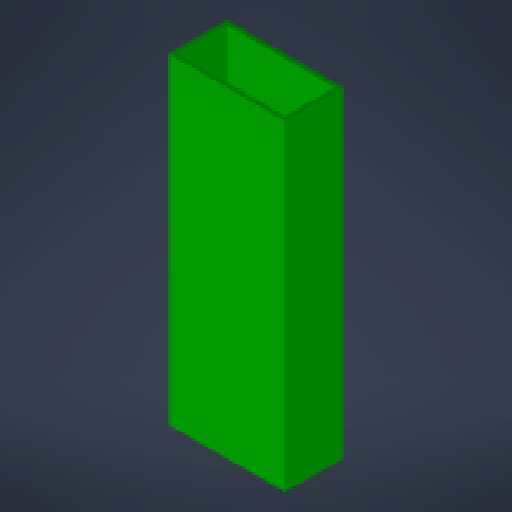
# Autodesk Inventor part: main axis
Saved by Autodesk Inventor 2024 (Build 280153000, 153)
## iProperties
Created: 2023-04-17
Part Number: main axis
Material: Типовые
Document SubType Name: Modeling
Designer: user
Density: 1 g/cm^3
Appearance: По умолчанию
Author: user
Autodesk Inventor part; units mm, degrees
ref_plane "YZ Plane" through (0, 0, 0) normal (1, 0, 0) x (0, 1, 0)
ref_plane "XZ Plane" through (0, 0, 0) normal (0, 1, 0) x (-1, 0, 0)
ref_plane "XY Plane" through (0, 0, 0) normal (0, 0, 1) x (1, 0, 0)
sketch "Эскиз1" plane through (0, 0, 0) normal (0, 0, 1) x (1, 0, 0)
  line L0 (0, 0) -> (-40, 0)
  line L1 (-40, 0) -> (-40, 20)
  line L2 (-40, 20) -> (0, 20)
  line L3 (0, 20) -> (0, 0)
  line L4 (-1.5, 1.5) -> (-38.5, 1.5)
  line L5 (-38.5, 1.5) -> (-38.5, 18.5)
  line L6 (-38.5, 18.5) -> (-1.5, 18.5)
  line L7 (-1.5, 18.5) -> (-1.5, 1.5)
  point P0 (-20, 18.5)
  point P1 (-20, 20)
  point P2 (-38.5, 10)
  point P3 (-40, 10)
  dimension "d0" = 40
  dimension "d18" = 20
  dimension "d19" = 1.5
  dimension "d20" = 1.5
  constraints: 16 end point, 4 midpoint, 4 parallel, 2 horizontal, 2 perpendicular, 1 horizontal alignment, 1 vertical alignment
  measures "d0" distance of L1.end L2.end
  measures "d18" distance of L0.end L1.end
  measures "d19" horizontal distance of L1.end L5.end
  measures "d20" horizontal distance of L2.end L6.end
extrude "Выдавливание3" add sketch "Эскиз1" against normal blind 110
equation "\"d20\" = d19"
